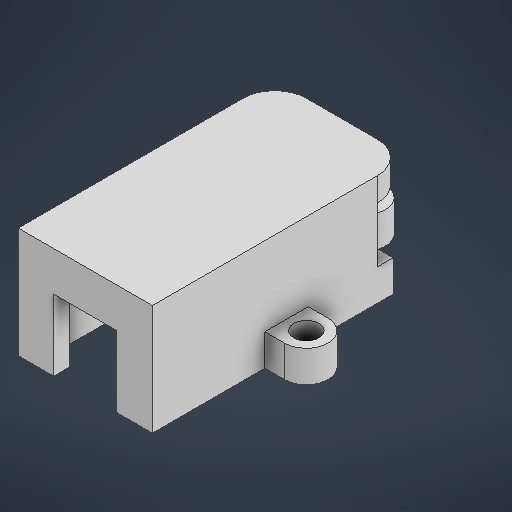
# Autodesk Inventor part: Część2-lewo
Saved by Autodesk Inventor 2026 (Build 300175000, 175)
## iProperties
Created: 2026-05-09
Part Number: Część2-lewo
Material: Ogólny
Document SubType Name: Modeling
Designer: Patryk Lombardo
Density: 1 g/cm^3
Appearance: Domyślna
Author: Patryk Lombardo
Autodesk Inventor part; units mm, degrees
ref_plane "YZ Plane" through (0, 0, 0) normal (1, 0, 0) x (0, 1, 0)
ref_plane "XZ Plane" through (0, 0, 0) normal (0, 1, 0) x (-1, 0, 0)
ref_plane "XY Plane" through (0, 0, 0) normal (0, 0, 1) x (1, 0, 0)
sketch "Szkic1" plane through (0, 0, 0) normal (0, 1, 0) x (-1, 0, 0)
  line L0 (0, 0) -> (0, -26.5) construction
  line L1 (6.5, -26.5) -> (-6.5, -26.5)
  line L2 (6.5, 0) -> (-6.5, 0)
  line L3 (-6.5, 0) -> (-6.5, 2)
  line L4 (-6.5, 2) -> (6.5, 2)
  line L5 (6.5, 2) -> (6.5, 0)
  line L6 (-6.5, 0) -> (-6.5, -10)
  line L7 (6.5, 0) -> (6.5, -10)
  line L8 (6.5, -10) -> (6.5, -26.5)
  line L9 (-6.5, -10) -> (-6.5, -26.5)
  line L10 (-6.5, 2) -> (-8.5, 2)
  line L11 (2, -26.5) -> (2, -30.5)
  line L12 (2, -30.5) -> (-2, -30.5)
  line L13 (-2, -30.5) -> (-2, -26.5)
  line L14 (-8.5, 2) -> (-8.5, -26.5)
  line L15 (-8.5, -26.5) -> (-6.5, -26.5)
  line L16 (6.5, -26.5) -> (8.5, -26.5)
  line L17 (8.5, -26.5) -> (8.5, 2)
  line L18 (8.5, 2) -> (6.5, 2)
  line L19 (11, -15) -> (-11, -15) construction
  circle A0 centre (-11, -15) radius 1.6
  circle A1 centre (11, -15) radius 1.6
  arc A2 (-11, -12.25) -> (-11, -17.75) centre (-11, -15) ccw
  arc A3 (11, -17.75) -> (11, -12.25) centre (11, -15) ccw
  line L20 (11, -12.25) -> (8.5, -12.25)
  line L21 (11, -17.75) -> (8.5, -17.75)
  line L22 (-11, -17.75) -> (-8.5, -17.75)
  line L23 (-11, -12.25) -> (-8.5, -12.25)
  line L24 (0, -30.5) -> (0, -33.25) construction
  circle A4 centre (0, -33.25) radius 1.6
  circle A5 centre (0, -33.25) radius 2.75
  line L25 (2, -30.5) -> (2, -31.3625)
  line L26 (-2, -30.5) -> (-2, -31.3625)
  line L27 (8.5, -26.5) -> (8.5, -28.5)
  line L28 (8.5, -28.5) -> (2, -28.5)
  line L29 (-8.5, -26.5) -> (-8.5, -28.5)
  line L30 (-8.5, -28.5) -> (-2, -28.5)
  point P0 (0, -15)
  dimension "d0" = 26.5
  dimension "d1" = 13
  dimension "d2" = 2
  dimension "d3" = 13
  dimension "d4" = 10
  dimension "d5" = 10
  dimension "d6" = 4
  dimension "d7" = 4
  dimension "d8" = 4.5
  dimension "d9" = 2
  dimension "d10" = 2
  dimension "d11" = 22
  dimension "d12" = 3.2
  dimension "d13" = 3.2
  dimension "d14" = 5.5
  dimension "d15" = 5.5
  dimension "d16" = 15
  dimension "d33" = 2.75
  dimension "d34" = 3.2
  dimension "d35" = 2
  dimension "d36" = 2
  constraints: 62 end point, 10 perpendicular, 10 point on line, 10 vertical, 8 midpoint, 7 point on circle, 6 centre point, 6 coincident, 4 horizontal, 2 parallel, 2 tangent
  measures "d0" distance of L0.start L0.end
  measures "d1" distance of L1.start L1.end
  measures "d2" distance of L4.end L2.start
  measures "d3" distance of L3.end L4.end
  measures "d4" distance of L2.start L7.end
  measures "d5" distance of L2.end L6.end
  measures "d6" distance of L11.start L11.end
  measures "d7" distance of L11.end L12.end
  measures "d8" distance from line of L1.end L13
  measures "d9" distance of L1.start L16.end
  measures "d10" distance of L14.end L1.end
  measures "d11" distance of L19.start L19.end
  measures "d12" diameter of A1
  measures "d13" diameter of A0
  measures "d14" diameter of A3
  measures "d15" diameter of A2
  measures "d16" distance between parallel lines of L2 L19
  measures "d33" distance of L24.start L24.end
  measures "d34" diameter of A4
  measures "d35" distance of L14.end L29.end
  measures "d36" distance of L16.end L27.end
extrude "Wyciągnięcie proste1" add sketch "Szkic1" along normal blind 11 contours L8 L7 L5 L18 L17 L16 | L11 L12 L13 L1 | L2 L3 L4 L5 | L15 L14 L10 L3 L6 L9
extrude "Wyciągnięcie proste2" add sketch "Szkic1" along normal blind 4 contours L16 L27 L28 L11 L1 | L13 L30 L29 L15 L1 | A5 | L22 A2 L23 L14
sketch "Szkic2" plane through (0, 11, 0) normal (0, 1, 0) x (1, 0, 0)
  line L0 (0, 0) -> (-8.5, 0)
  line L1 (-8.5, 0) -> (-8.5, 30.5)
  line L2 (-8.5, 30.5) -> (8.5, 30.5)
  line L3 (8.5, 30.5) -> (8.5, -2)
  line L4 (8.5, -2) -> (-8.5, -2)
  line L5 (-8.5, -2) -> (-8.5, 0)
  dimension "d21" = 8.5
  dimension "d22" = 17
  dimension "d23" = 32.5
  dimension "d24" = 2
  constraints: 12 end point, 5 perpendicular, 1 horizontal, 1 point on line
  measures "d21" distance of L0.start L0.end
  measures "d22" distance of L1.end L2.end
  measures "d23" distance between parallel lines of L4 L2
  measures "d24" distance between parallel lines of L4 L0
extrude "Wyciągnięcie proste3" add sketch "Szkic2" along normal blind 3
fillet "Zaokrąglenie1" radius 4 2 edges at (8.5, 12.5, -30.5) (-8.5, 12.5, -30.5)
sketch "Szkic3" plane through (-8.5, 0, 2) normal (0, 0, 1) x (1, 0, 0)
  line L0 (0, 0) -> (8.5, 0) construction
  line L1 (4.5, 0) -> (12.5, 0)
  line L2 (4.5, 0) -> (4.5, 9)
  line L3 (4.5, 9) -> (12.5, 9)
  line L4 (12.5, 9) -> (12.5, 0)
  dimension "d28" = 8.5
  dimension "d29" = 8
  dimension "d30" = 9
  constraints: 10 end point, 2 horizontal, 2 perpendicular, 1 midpoint, 1 vertical
  measures "d28" distance of L0.start L0.end
  measures "d29" distance of L1.start L1.end
  measures "d30" distance of L3.end L1.end
extrude "Wyciągnięcie proste4" cut sketch "Szkic3" against normal blind 3
equation "\"d3\" = d1"
equation "\"d5\" = d4"
equation "\"d10\" = d9"
